Autodesk Inventor part; units mm, degrees
(part 2 of 2)
sketch "Sketch40" plane through (-6.2022, 0, 0) normal (0, 0, -1) x (-1, 0, 0)
  circle A0 centre (0, 0) radius 3.5 construction
  arc A1 (4.4538, 8.9534) -> (7.9648, -6.0466) centre (0, 0) ccw construction
  line L0 (7.9648, -6.0466) -> (20.9538, -6.0466) construction
  line L1 (20.9538, -6.0466) -> (20.9538, 8.9534) construction
  line L2 (20.9538, 8.9534) -> (4.4538, 8.9534) construction
  line L3 (20.9538, 8.9534) -> (10.9538, 8.9534)
  line L4 (10.9538, 8.9534) -> (10.9538, 2.9534)
  line L5 (10.9538, 2.9534) -> (20.9538, 2.9534)
  line L6 (20.9538, 2.9534) -> (20.9538, 8.9534)
  point P0 (-6.2022, 0)
  dimension "d201" = 10
  dimension "d202" = 6
  constraints: 8 end point, 2 parallel, 1 horizontal, 1 perpendicular
  measures "d201" distance of L5.end L4.end
  measures "d202" distance of L4.end L3.end
extrude "Extrusion30" add sketch "Sketch40" along normal blind 20
sketch "Sketch41" plane through (-27.156, 2.9534, 0) normal (0, -1, 0) x (1, 0, 0)
  line L0 (0, 0) -> (10, 0) projected
  line L1 (0, 0) -> (0, -20) projected
  line L2 (10, -20) -> (0, -20) projected
  line L3 (10, 0) -> (10, -20) projected
  line L4 (10, -20) -> (0, -20) projected
  line L5 (5, -20) -> (5, 0)
  line L6 (0, 0) -> (10, 0) projected
  line L7 (10, 0) -> (10, -20) projected
  line L8 (10, -10) -> (0, -10)
  point P0 (27.156, 0)
  point P1 (5, -15)
  point P2 (5, -5)
  dimension "d205" = 10
  dimension "d206" = 5
  dimension "d207" = 5
  constraints: 4 end point, 4 midpoint, 2 point on line
  measures "d205" distance between parallel lines of L8 L2
  measures "d206" distance from line of L2 point (5, -15)
  measures "d207" distance from line of L8 point (5, -5)
hole "Hole4" at (-22.156, 2.9534, -15) at (-22.156, 2.9534, -5) direction (0, 1, 0) diameter 5 end through all countersink diameter 7 countersink angle 90
fillet "Fillet11" radius 2 1 edges at (-22.156, 2.9534, 0)
fillet "Fillet12" radius 2 1 edges at (-17.156, 4.9534, 0)
sketch "Sketch44" plane through (-6.2022, 0, 0) normal (0, 0, -1) x (-1, 0, 0)
  line L0 (10.4, -11.325) -> (10.4, 7.925) construction
  line L1 (-15.85, -11.325) -> (10.4, -11.325) construction
  circle A0 centre (-11.35, -8.625) radius 1.5 construction
  circle A1 centre (5.9, -8.625) radius 1.5 construction
  line L2 (-15.85, 7.925) -> (-15.85, -11.325) construction
  line L3 (20.9538, -6.0466) -> (7.9648, -6.0466) projected
  line L4 (10.4, -6.0466) -> (-15.85, -6.0466)
  line L5 (-15.85, -6.0466) -> (-15.85, -11.325)
  line L6 (-15.85, -11.325) -> (10.4, -11.325)
  line L7 (10.4, -11.325) -> (10.4, -6.0466)
  point P0 (-6.2022, 0)
  constraints: 8 end point, 2 parallel, 2 point on line, 1 horizontal, 1 perpendicular
extrude "Extrusion32" add sketch "Sketch44" against normal blind 4
sketch "Sketch45" plane through (-6.2022, 0, 0) normal (0, 0, -1) x (-1, 0, 0)
  circle A0 centre (-11.35, -8.625) radius 1.5 construction
  circle A1 centre (5.9, -8.625) radius 1.5 construction
  circle A2 centre (-11.35, -8.625) radius 2.5
  circle A3 centre (5.9, -8.625) radius 2.5
  point P0 (-6.2022, 0)
  dimension "d225" = 5
  dimension "d226" = 5
  constraints: 2 centre point, 2 coincident
  measures "d225" diameter of A2
  measures "d226" diameter of A3
thicken "Thicken17" operation add thickness 1 both sides no extend neighbours yes toward (0, 1, 0) faces at (7.0194, -6.0466, 1.3333)
thicken "Thicken18" operation add thickness 1 both sides no extend neighbours yes toward (0, -1, 0) faces at (-7.8522, -11.325, 1.3333)
extrude "Extrusion33" add sketch "Sketch45" along normal blind 6.7
sketch "Sketch46" plane through (5.1478, -8.625, -6.7) normal (0, 0, -1) x (-1, 0, 0)
  circle A0 centre (0, 0) radius 2.5 projected
  circle A1 centre (17.25, 0) radius 2.5 projected
  point P0 (5.1478, 8.625)
  constraints: 2 coincident
hole "Hole5" at (5.1478, -8.625, -6.7) at (-12.1022, -8.625, -6.7) direction (0, 0, 1) diameter 3 end through all
fillet "Fillet13" radius 2 8 edges at (2.431, -5.0466, 2) (9.6478, -12.325, 2) (9.6478, -5.0466, 2) (-16.6022, -12.325, 2) (-16.6022, -6.0466, 2) (-27.156, -6.0466, 2) (-27.156, 5.9534, -20) (-17.156, 5.9534, -20)
sketch "Sketch42" plane through (-6.2022, 0, 0) normal (0, 0, -1) x (-1, 0, 0)
  line L0 (-10, 14.2035) -> (10, 14.2035)
  line L1 (10, 14.2035) -> (10, 8.2035)
  line L2 (10, 8.2035) -> (-10, 8.2035)
  line L3 (-10, 8.2035) -> (-10, 14.2035)
  line L4 (0, 11.2163) -> (0, -11.325) construction
  point P0 (-6.2022, 0)
  dimension "d217" = 20
  dimension "d218" = 6
  dimension "d219" = 10
  dimension "d222" = 1.2
  constraints: 8 end point, 1 perpendicular, 1 other
  measures "d222" distance between parallel lines of L1 L4
body "Solid1"
